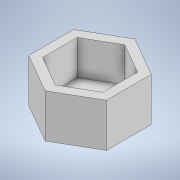
# Autodesk Inventor part: Improved Internal Base
Saved by Autodesk Inventor 2020 (Build 240168000, 168)
## iProperties
Created: 2020-02-13
Part Number: Improved Internal Base
Material: Generic
Document SubType Name: Modeling
Designer: danie
Density: 1 g/cm^3
Appearance: Default
Author: danie
Autodesk Inventor part; units mm, degrees
ref_plane "YZ Plane" through (0, 0, 0) normal (1, 0, 0) x (0, 1, 0)
ref_plane "XZ Plane" through (0, 0, 0) normal (0, 1, 0) x (-1, 0, 0)
ref_plane "XY Plane" through (0, 0, 0) normal (0, 0, 1) x (1, 0, 0)
sketch "Sketch1" plane through (0, 0, 0) normal (0, 1, 0) x (-1, 0, 0)
  line L0 (0, 0) -> (0, -80)
  line L1 (0, -80) -> (69.282, -120)
  line L2 (69.282, -120) -> (138.5641, -80)
  line L3 (138.5641, -80) -> (138.5641, 0)
  line L4 (138.5641, 0) -> (69.282, 40)
  line L5 (69.282, 40) -> (0, 0)
  line L6 (-20, 11.547) -> (-20, -91.547)
  line L7 (-20, -91.547) -> (69.282, -143.094)
  line L8 (69.282, -143.094) -> (158.5641, -91.547)
  line L9 (158.5641, -91.547) -> (158.5641, 11.547)
  line L10 (158.5641, 11.547) -> (69.282, 63.094)
  line L11 (69.282, 63.094) -> (-20, 11.547)
  line L12 (0, 0) -> (-20, 0) construction
  line L13 (-20, 11.547) -> (0, 0) construction
  dimension "innerWall" = 80
  dimension "d1" = 80
  dimension "d2" = 80
  dimension "d3" = 80
  dimension "d4" = 80
  dimension "d5" = 80
  dimension "d6" = 120
  dimension "d7" = 120
  dimension "d9" = 120
  dimension "d10" = 120
  dimension "d11" = 120
  dimension "wallThickness" = 20
  dimension "d15" = 20
  dimension "d16" = 178.5641
  constraints: 28 end point, 5 equal length, 2 vertical, 1 parallel, 1 perpendicular, 1 point on line
  measures "innerWall" distance of L0.start L0.end
  measures "d1" distance of L0.end L1.end
  measures "d2" distance of L1.end L2.end
  measures "d3" distance of L2.end L3.end
  measures "d4" distance of L3.end L4.end
  measures "d5" distance of L0.start L4.end
  measures "d6" angle of L0 L1
  measures "d7" angle of L1 L2
  measures "d9" angle of L2 L3
  measures "d10" angle of L6 L7
  measures "d11" angle of L7 L8
  measures "wallThickness" distance between parallel lines of L6 L0
  measures "d15" distance between parallel lines of L11 L5
  measures "d16" horizontal distance of L6.start L8.end
extrude "Extrusion1" add sketch "Sketch1" along normal blind 20 contours L5 L4 L3 L2 L1 L0
extrude "Extrusion2" add sketch "Sketch1" along normal blind 100
equation "\"d1\" = innerWall"
equation "\"d2\" = innerWall"
equation "\"d3\" = innerWall"
equation "\"d4\" = innerWall"
equation "\"d5\" = innerWall"
body "Solid1"
